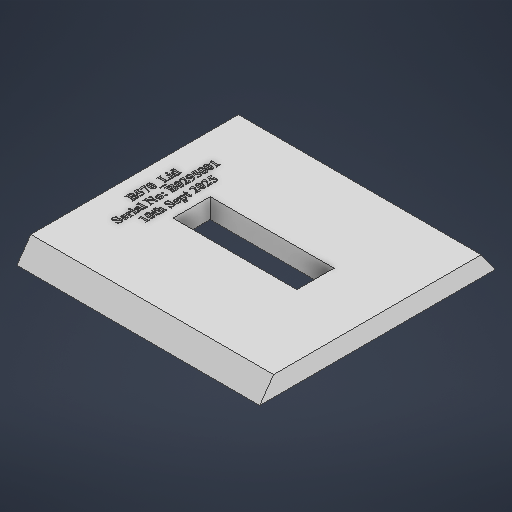
# Autodesk Inventor part: Lid_295
Saved by Autodesk Inventor 2026.1 (Build 301233000, 233)
## iProperties
Created: 2025-09-11
Part Number: Lid_295
Material: Generic
Document SubType Name: Modeling
Designer: usman
Density: 1 g/cm^3
Appearance: Default
Author: usman
Autodesk Inventor part; units mm, degrees
(part 1 of 2)
ref_plane "YZ Plane" through (0, 0, 0) normal (1, 0, 0) x (0, 1, 0)
ref_plane "XZ Plane" through (0, 0, 0) normal (0, 1, 0) x (-1, 0, 0)
ref_plane "XY Plane" through (0, 0, 0) normal (0, 0, 1) x (1, 0, 0)
sketch "Sketch1" plane through (0, 0, 0) normal (1, 0, 0) x (0, 1, 0)
  line L0 (-4, 47.5) -> (4, 47.5)
  line L1 (4, 47.5) -> (4, -47.5)
  line L2 (4, -47.5) -> (-4, -47.5)
  line L3 (-4, -47.5) -> (-4, 47.5)
  line L4 (-4, 47.5) -> (4, -47.5) construction
  line L5 (4, 47.5) -> (-4, -47.5) construction
  line L6 (-4, 47.5) -> (4, 41.8983)
  line L7 (-4, -47.5) -> (4, -41.8983)
  point P0 (0, 0)
  dimension "d0" = 95
  dimension "d1" = 8
  dimension "d2" = 125
  dimension "d3" = 125
  constraints: 16 end point, 2 midpoint, 2 parallel, 2 point on line, 1 horizontal, 1 perpendicular
  measures "d0" distance of L2.end L0.start
  measures "d1" distance of L1.end L2.end
  measures "d2" angle of L1 L6
  measures "d3" angle of L1 L7
extrude "Extrusion1" add sketch "Sketch1" along normal blind 98 contours L6 L1 L7 L3
sketch "Sketch2" plane through (0, 4, 41.8983) normal (0, 1, 0) x (1, 0, 0)
  line L0 (-3.8878, 0.5072) -> (-3.8878, 83.7387) construction
  line L1 (-3.8878, 83.7387) -> (29.5232, 83.7387) construction
  line L2 (29.5232, 83.7387) -> (29.5232, 0.5072) construction
  line L3 (29.5232, 0.5072) -> (-3.8878, 0.5072) construction
  spline S0 degree 2 poles (7.224, 34.2529) (7.3303, 34.7069) (7.4808, 34.891) knots 0 0 0 1 1 1
  spline S1 degree 2 poles (7.4808, 34.891) (7.6935, 35.1556) (8.0333, 35.1556) knots 0 0 0 1 1 1
  spline S2 degree 2 poles (8.0333, 35.1556) (8.3913, 35.1556) (8.6247, 34.8677) knots 0 0 0 1 1 1
  spline S3 degree 2 poles (8.6247, 34.8677) (8.9075, 34.5149) (8.9075, 33.8405) knots 0 0 0 1 1 1
  line L4 (8.9075, 33.8405) -> (8.9075, 32.2244)
  line L5 (8.9075, 32.2244) -> (8.8219, 32.2244)
  spline S4 degree 2 poles (8.8219, 32.2244) (8.8219, 32.4449) (8.7389, 32.6032) (8.6092, 32.6654) (8.3498, 32.6654) knots 0 0 0 1 2 3 3 3
  line L6 (8.3498, 32.6654) -> (6.2902, 32.6654)
  spline S5 degree 2 poles (6.2902, 32.6654) (6.0308, 32.6654) (5.8985, 32.6032) (5.8181, 32.4449) (5.8181, 32.2244) knots 0 0 0 1 2 3 3 3
  line L7 (5.8181, 32.2244) -> (5.7325, 32.2244)
  line L8 (5.7325, 32.2244) -> (5.7325, 33.7471)
  spline S6 degree 2 poles (5.7325, 33.7471) (5.7325, 34.2944) (5.927, 34.7484) (6.3135, 35.0103) (6.5314, 35.0103) knots 0 0 0 1 2 3 3 3
  spline S7 degree 2 poles (6.5314, 35.0103) (6.7597, 35.0103) (7.1202, 34.6757) (7.224, 34.2529) knots 0 0 0 1 2 2 2
  line L9 (7.3433, 33.4047) -> (8.3627, 33.4047)
  line L10 (8.3627, 33.4047) -> (8.4769, 33.4021)
  spline S8 degree 2 poles (8.4769, 33.4021) (8.604, 33.4021) (8.7311, 33.5292) (8.7311, 33.6537) knots 0 0 0 1 2 2 2
  spline S9 degree 2 poles (8.7311, 33.6537) (8.7311, 33.8353) (8.5651, 34.144) (8.2486, 34.31) (8.0567, 34.31) knots 0 0 0 1 2 3 3 3
  spline S10 degree 2 poles (8.0567, 34.31) (7.8336, 34.31) (7.4808, 34.1258) (7.3407, 33.7652) (7.3433, 33.4047) knots 0 0 0 1 2 3 3 3
  spline S11 degree 2 poles (7.1617, 33.4047) (7.1617, 33.7393) (7.0113, 34.0558) (6.7389, 34.2244) (6.5288, 34.2244) knots 0 0 0 1 2 3 3 3
  spline S12 degree 2 poles (6.5288, 34.2244) (6.3161, 34.2244) (6.0463, 34.0584) (5.9063, 33.7471) (5.9089, 33.4047) knots 0 0 0 1 2 3 3 3
  line L11 (5.9089, 33.4047) -> (7.1617, 33.4047)
  line L12 (5.7325, 36.0531) -> (5.7325, 37.5446)
  line L13 (5.7325, 37.5446) -> (6.3369, 37.3086)
  line L14 (6.3369, 37.3086) -> (6.3369, 36.0531)
  line L15 (6.3369, 36.0531) -> (6.6533, 35.9364)
  spline S13 degree 2 poles (6.6533, 35.9364) (6.6845, 36.7457) (7.0554, 37.1815) knots 0 0 0 1 1 1
  spline S14 degree 2 poles (7.0554, 37.1815) (7.3615, 37.5395) (7.818, 37.5395) knots 0 0 0 1 1 1
  spline S15 degree 2 poles (7.818, 37.5395) (8.1111, 37.5395) (8.6714, 37.2074) (8.9723, 36.603) (8.9723, 36.2399) knots 0 0 0 1 2 3 3 3
  spline S16 degree 2 poles (8.9723, 36.2399) (8.9723, 35.8508) (8.8271, 35.6433) knots 0 0 0 1 1 1
  spline S17 degree 2 poles (8.8271, 35.6433) (8.7233, 35.498) (8.5936, 35.498) knots 0 0 0 1 1 1
  spline S18 degree 2 poles (8.5936, 35.498) (8.4924, 35.498) (8.3368, 35.6511) (8.3368, 35.7522) knots 0 0 0 1 2 2 2
  spline S19 degree 2 poles (8.3368, 35.7522) (8.3368, 35.843) (8.412, 36.0298) (8.5728, 36.258) knots 0 0 0 1 2 2 2
  spline S20 degree 2 poles (8.5728, 36.258) (8.6714, 36.4007) (8.7077, 36.5045) knots 0 0 0 1 1 1
  spline S21 degree 2 poles (8.7077, 36.5045) (8.7363, 36.5771) (8.7363, 36.6679) knots 0 0 0 1 1 1
  spline S22 degree 2 poles (8.7363, 36.6679) (8.7363, 36.8598) (8.4561, 37.1296) (8.259, 37.1296) knots 0 0 0 1 2 2 2
  spline S23 degree 2 poles (8.259, 37.1296) (7.8465, 37.1296) (7.3329, 36.3047) (7.3329, 35.6744) knots 0 0 0 1 2 2 2
  spline S24 degree 2 poles (7.3329, 35.6744) (7.3329, 35.6121) (7.3355, 35.485) knots 0 0 0 1 1 1
  line L16 (7.3355, 35.485) -> (5.7325, 36.0531)
  line L17 (8.9723, 38.5744) -> (6.3524, 39.4382)
  line L18 (6.3524, 39.4382) -> (6.3524, 38.7794)
  spline S25 degree 2 poles (6.3524, 38.7794) (6.3524, 38.3929) (6.4536, 38.1983) knots 0 0 0 1 1 1
  spline S26 degree 2 poles (6.4536, 38.1983) (6.5236, 38.0634) (6.7182, 37.9726) knots 0 0 0 1 1 1
  line L19 (6.7182, 37.9726) -> (6.7182, 37.8844)
  line L20 (6.7182, 37.8844) -> (5.7325, 38.1153)
  line L21 (5.7325, 38.1153) -> (5.7325, 40.0115)
  line L22 (5.7325, 40.0115) -> (8.9723, 38.9428)
  line L23 (8.9723, 38.9428) -> (8.9723, 38.5744)
  spline S27 degree 2 poles (7.32, 42.346) (7.7947, 42.346) (8.2071, 42.2138) knots 0 0 0 1 1 1
  spline S28 degree 2 poles (8.2071, 42.2138) (8.4587, 42.1333) (8.783, 41.8636) (8.9723, 41.5212) (8.9723, 41.3214) knots 0 0 0 1 2 3 3 3
  spline S29 degree 2 poles (8.9723, 41.3214) (8.9723, 41.0906) (8.7389, 40.7196) (8.521, 40.577) knots 0 0 0 1 2 2 2
  spline S30 degree 2 poles (8.521, 40.577) (8.3627, 40.4758) (8.0982, 40.398) knots 0 0 0 1 1 1
  spline S31 degree 2 poles (8.0982, 40.398) (7.7376, 40.2968) (7.3563, 40.2968) knots 0 0 0 1 1 1
  spline S32 degree 2 poles (7.3563, 40.2968) (6.8401, 40.2968) (6.4069, 40.4421) knots 0 0 0 1 1 1
  spline S33 degree 2 poles (6.4069, 40.4421) (6.0489, 40.5614) (5.6676, 41.0491) (5.6676, 41.3214) knots 0 0 0 1 2 2 2
  spline S34 degree 2 poles (5.6676, 41.3214) (5.6676, 41.5964) (6.0437, 42.0763) (6.3628, 42.1904) knots 0 0 0 1 2 2 2
  spline S35 degree 2 poles (6.3628, 42.1904) (6.8012, 42.346) (7.32, 42.346) knots 0 0 0 1 1 1
  spline S36 degree 2 poles (7.3148, 41.6249) (6.4821, 41.6249) (6.3446, 41.6146) knots 0 0 0 1 1 1
  spline S37 degree 2 poles (6.3446, 41.6146) (6.0178, 41.5912) (5.9037, 41.503) knots 0 0 0 1 1 1
  spline S38 degree 2 poles (5.9037, 41.503) (5.8284, 41.4459) (5.8284, 41.3137) knots 0 0 0 1 1 1
  spline S39 degree 2 poles (5.8284, 41.3137) (5.8284, 41.2125) (5.8855, 41.1554) knots 0 0 0 1 1 1
  spline S40 degree 2 poles (5.8855, 41.1554) (5.9659, 41.0672) (6.381, 41.0076) (7.6183, 41.0076) knots 0 0 0 1 2 2 2
  spline S41 degree 2 poles (7.6183, 41.0076) (8.2927, 41.0076) (8.5236, 41.0543) knots 0 0 0 1 1 1
  spline S42 degree 2 poles (8.5236, 41.0543) (8.6896, 41.0906) (8.8011, 41.2203) (8.8011, 41.3292) knots 0 0 0 1 2 2 2
  spline S43 degree 2 poles (8.8011, 41.3292) (8.8011, 41.4459) (8.7259, 41.503) knots 0 0 0 1 1 1
  spline S44 degree 2 poles (8.7259, 41.503) (8.5962, 41.6016) (8.3212, 41.6146) knots 0 0 0 1 1 1
  line L24 (8.3212, 41.6146) -> (7.3148, 41.6249)
  line L25 (9.6364, 42.4783) -> (9.6364, 44.9659)
  line L26 (9.6364, 44.9659) -> (9.9425, 44.9659)
  line L27 (9.9425, 44.9659) -> (9.9425, 42.4783)
  line L28 (9.9425, 42.4783) -> (9.6364, 42.4783)
  line L29 (7.7921, 47.949) -> (8.9075, 47.8297)
  line L30 (8.9075, 47.8297) -> (8.9075, 45.0126)
  line L31 (8.9075, 45.0126) -> (8.8219, 45.0126)
  line L32 (8.8219, 45.0126) -> (8.8219, 45.119)
  spline S45 degree 2 poles (8.8219, 45.119) (8.8219, 45.2565) (8.7726, 45.3395) knots 0 0 0 1 1 1
  spline S46 degree 2 poles (8.7726, 45.3395) (8.7389, 45.3991) (8.661, 45.4329) knots 0 0 0 1 1 1
  spline S47 degree 2 poles (8.661, 45.4329) (8.604, 45.4588) (8.3653, 45.4588) knots 0 0 0 1 1 1
  line L33 (8.3653, 45.4588) -> (6.2746, 45.4588)
  spline S48 degree 2 poles (6.2746, 45.4588) (6.0308, 45.4588) (5.9089, 45.4069) (5.8181, 45.2513) (5.8181, 45.119) knots 0 0 0 1 2 3 3 3
  line L34 (5.8181, 45.119) -> (5.8181, 45.0126)
  line L35 (5.8181, 45.0126) -> (5.7325, 45.0126)
  line L36 (5.7325, 45.0126) -> (5.7325, 46.7039)
  line L37 (5.7325, 46.7039) -> (5.8181, 46.7039)
  line L38 (5.8181, 46.7039) -> (5.8181, 46.5664)
  spline S49 degree 2 poles (5.8181, 46.5664) (5.8181, 46.4263) (5.8674, 46.3433) knots 0 0 0 1 1 1
  spline S50 degree 2 poles (5.8674, 46.3433) (5.9011, 46.2811) (5.9789, 46.2474) knots 0 0 0 1 1 1
  spline S51 degree 2 poles (5.9789, 46.2474) (6.036, 46.2214) (6.2746, 46.2214) knots 0 0 0 1 1 1
  line L39 (6.2746, 46.2214) -> (8.2979, 46.2214)
  spline S52 degree 2 poles (8.2979, 46.2214) (8.5417, 46.2214) (8.674, 46.2785) (8.7077, 46.3589) knots 0 0 0 1 2 2 2
  spline S53 degree 2 poles (8.7077, 46.3589) (8.7285, 46.4186) (8.7285, 46.6416) knots 0 0 0 1 1 1
  line L40 (8.7285, 46.6416) -> (8.7285, 46.9062)
  spline S54 degree 2 poles (8.7285, 46.9062) (8.7285, 47.1604) (8.5495, 47.4976) (8.1656, 47.7441) (7.7921, 47.853) knots 0 0 0 1 2 3 3 3
  line L41 (7.7921, 47.853) -> (7.7921, 47.949)
  line L42 (6.7182, 49.137) -> (8.4535, 49.137)
  spline S55 degree 2 poles (8.4535, 49.137) (8.687, 49.137) (8.8141, 49.246) (8.8245, 49.4042) knots 0 0 0 1 2 2 2
  line L43 (8.8245, 49.4042) -> (8.9075, 49.4042)
  line L44 (8.9075, 49.4042) -> (8.9075, 48.2188)
  line L45 (8.9075, 48.2188) -> (8.8245, 48.2188)
  spline S56 degree 2 poles (8.8245, 48.2188) (8.8193, 48.364) (8.7389, 48.4341) knots 0 0 0 1 1 1
  spline S57 degree 2 poles (8.7389, 48.4341) (8.687, 48.4807) (8.4535, 48.4807) knots 0 0 0 1 1 1
  line L46 (8.4535, 48.4807) -> (7.1747, 48.4807)
  spline S58 degree 2 poles (7.1747, 48.4807) (6.9413, 48.4807) (6.8141, 48.3744) (6.8038, 48.2188) knots 0 0 0 1 2 2 2
  line L47 (6.8038, 48.2188) -> (6.7182, 48.2188)
  line L48 (6.7182, 48.2188) -> (6.7182, 49.137)
  spline S59 degree 2 poles (5.6598, 48.8102) (5.6598, 48.9632) (5.8725, 49.1733) (6.023, 49.1733) knots 0 0 0 1 2 2 2
  spline S60 degree 2 poles (6.023, 49.1733) (6.1734, 49.1733) (6.3836, 48.9606) (6.3836, 48.8102) knots 0 0 0 1 2 2 2
  spline S61 degree 2 poles (6.3836, 48.8102) (6.3836, 48.6597) (6.1734, 48.4496) (6.023, 48.4496) knots 0 0 0 1 2 2 2
  spline S62 degree 2 poles (6.023, 48.4496) (5.8725, 48.4496) (5.6598, 48.6597) (5.6598, 48.8102) knots 0 0 0 1 2 2 2
  line L49 (5.7325, 51.7439) -> (8.2512, 51.7439)
  spline S63 degree 2 poles (8.2512, 51.7439) (8.508, 51.7439) (8.5547, 51.7569) knots 0 0 0 1 1 1
  spline S64 degree 2 poles (8.5547, 51.7569) (8.6299, 51.7777) (8.7051, 51.8814) (8.7155, 52.0111) knots 0 0 0 1 2 2 2
  line L50 (8.7155, 52.0111) -> (8.7933, 52.0111)
  line L51 (8.7933, 52.0111) -> (8.9723, 51.0877)
  line L52 (8.9723, 51.0877) -> (8.6247, 51.0877)
  spline S65 degree 2 poles (8.6247, 51.0877) (8.8271, 50.9217) (8.9723, 50.6623) (8.9723, 50.4963) knots 0 0 0 1 2 2 2
  spline S66 degree 2 poles (8.9723, 50.4963) (8.9723, 50.0786) (8.5988, 49.8348) knots 0 0 0 1 1 1
  spline S67 degree 2 poles (8.5988, 49.8348) (8.2927, 49.6377) (7.8517, 49.6377) knots 0 0 0 1 1 1
  spline S68 degree 2 poles (7.8517, 49.6377) (7.499, 49.6377) (6.9387, 49.8815) (6.6533, 50.3043) (6.6533, 50.5481) knots 0 0 0 1 2 3 3 3
  spline S69 degree 2 poles (6.6533, 50.5481) (6.6533, 50.7064) (6.7752, 50.9502) (6.9283, 51.0877) knots 0 0 0 1 2 2 2
  line L53 (6.9283, 51.0877) -> (6.2668, 51.0877)
  spline S70 degree 2 poles (6.2668, 51.0877) (6.0152, 51.0877) (5.9633, 51.0669) knots 0 0 0 1 1 1
  spline S71 degree 2 poles (5.9633, 51.0669) (5.8959, 51.0384) (5.831, 50.9268) (5.831, 50.7712) knots 0 0 0 1 2 2 2
  line L54 (5.831, 50.7712) -> (5.7325, 50.7712)
  line L55 (5.7325, 50.7712) -> (5.7325, 51.7439)
  spline S72 degree 2 poles (7.2188, 51.0877) (6.8842, 50.9139) (6.8842, 50.6649) knots 0 0 0 1 1 1
  spline S73 degree 2 poles (6.8842, 50.6649) (6.8842, 50.5767) (6.9309, 50.5222) knots 0 0 0 1 1 1
  spline S74 degree 2 poles (6.9309, 50.5222) (7.0035, 50.434) (7.3693, 50.3251) (7.7454, 50.3251) knots 0 0 0 1 2 2 2
  spline S75 degree 2 poles (7.7454, 50.3251) (8.1604, 50.3251) (8.5599, 50.447) (8.6481, 50.5507) knots 0 0 0 1 2 2 2
  spline S76 degree 2 poles (8.6481, 50.5507) (8.6922, 50.6052) (8.6922, 50.6986) knots 0 0 0 1 1 1
  spline S77 degree 2 poles (8.6922, 50.6986) (8.6922, 50.9061) (8.3705, 51.0877) knots 0 0 0 1 1 1
  line L56 (8.3705, 51.0877) -> (7.2188, 51.0877)
  line L57 (10.6816, 23.453) -> (11.7399, 23.4789)
  line L58 (11.7399, 23.4789) -> (11.7399, 23.3829)
  spline S78 degree 2 poles (11.7399, 23.3829) (11.343, 23.3155) (10.8579, 22.7811) (10.8579, 22.4725) knots 0 0 0 1 2 2 2
  spline S79 degree 2 poles (10.8579, 22.4725) (10.8579, 22.2338) (11.1121, 21.9537) (11.2782, 21.9537) knots 0 0 0 1 2 2 2
  spline S80 degree 2 poles (11.2782, 21.9537) (11.3845, 21.9537) (11.4649, 22.003) knots 0 0 0 1 1 1
  spline S81 degree 2 poles (11.4649, 22.003) (11.5765, 22.0704) (11.6828, 22.2209) knots 0 0 0 1 1 1
  spline S82 degree 2 poles (11.6828, 22.2209) (11.7606, 22.3324) (11.9578, 22.7319) knots 0 0 0 1 1 1
  spline S83 degree 2 poles (11.9578, 22.7319) (12.2301, 23.2896) (12.474, 23.4841) knots 0 0 0 1 1 1
  spline S84 degree 2 poles (12.474, 23.4841) (12.7178, 23.6761) (13.0317, 23.6761) knots 0 0 0 1 1 1
  spline S85 degree 2 poles (13.0317, 23.6761) (13.4286, 23.6761) (14.0018, 23.0561) (14.0018, 22.5762) knots 0 0 0 1 2 2 2
  spline S86 degree 2 poles (14.0018, 22.5762) (14.0018, 22.4258) (13.9422, 22.1586) (13.8566, 21.9589) knots 0 0 0 1 2 2 2
  spline S87 degree 2 poles (13.8566, 21.9589) (13.8099, 21.8447) (13.8099, 21.7721) knots 0 0 0 1 1 1
  spline S88 degree 2 poles (13.8099, 21.7721) (13.8099, 21.7124) (13.9058, 21.575) (14.0018, 21.5335) knots 0 0 0 1 2 2 2
  line L59 (14.0018, 21.5335) -> (14.0018, 21.4479)
  line L60 (14.0018, 21.4479) -> (12.8034, 21.4479)
  line L61 (12.8034, 21.4479) -> (12.8034, 21.5335)
  spline S89 degree 2 poles (12.8034, 21.5335) (13.3092, 21.6372) (13.8384, 22.226) (13.8384, 22.5658) knots 0 0 0 1 2 2 2
  spline S90 degree 2 poles (13.8384, 22.5658) (13.8384, 22.8278) (13.5531, 23.1391) (13.3637, 23.1391) knots 0 0 0 1 2 2 2
  spline S91 degree 2 poles (13.3637, 23.1391) (13.2522, 23.1391) (13.0395, 23.0198) (12.8501, 22.776) (12.6996, 22.4647) knots 0 0 0 1 2 3 3 3
  spline S92 degree 2 poles (12.6996, 22.4647) (12.4869, 22.0315) (12.186, 21.6528) (11.8177, 21.4504) (11.5946, 21.4504) knots 0 0 0 1 2 3 3 3
  spline S93 degree 2 poles (11.5946, 21.4504) (11.2159, 21.4504) (10.6816, 22.0081) (10.6816, 22.431) knots 0 0 0 1 2 2 2
  spline S94 degree 2 poles (10.6816, 22.431) (10.6816, 22.5866) (10.7179, 22.7319) knots 0 0 0 1 1 1
  spline S95 degree 2 poles (10.7179, 22.7319) (10.7464, 22.8408) (10.8994, 23.1573) (10.8994, 23.2221) knots 0 0 0 1 2 2 2
  spline S96 degree 2 poles (10.8994, 23.2221) (10.8994, 23.2818) (10.8242, 23.3518) (10.6816, 23.3829) knots 0 0 0 1 2 2 2
  line L62 (10.6816, 23.3829) -> (10.6816, 23.453)
  line L63 (12.7593, 25.8861) -> (12.7593, 24.6825)
  spline S97 degree 2 poles (12.7593, 24.6825) (13.1925, 24.7033) (13.4441, 24.916) knots 0 0 0 1 1 1
  spline S98 degree 2 poles (13.4441, 24.916) (13.6387, 25.0768) (13.6387, 25.3051) knots 0 0 0 1 1 1
  spline S99 degree 2 poles (13.6387, 25.3051) (13.6387, 25.4451) (13.483, 25.676) (13.2781, 25.8057) knots 0 0 0 1 2 2 2
  line L64 (13.2781, 25.8057) -> (13.33, 25.8861)
  spline S100 degree 2 poles (13.33, 25.8861) (13.6931, 25.7071) (13.994, 25.2765) (13.994, 24.9938) knots 0 0 0 1 2 2 2
  spline S101 degree 2 poles (13.994, 24.9938) (13.994, 24.5035) (13.6205, 24.2545) knots 0 0 0 1 1 1
  spline S102 degree 2 poles (13.6205, 24.2545) (13.317, 24.0522) (12.8709, 24.0522) knots 0 0 0 1 1 1
  spline S103 degree 2 poles (12.8709, 24.0522) (12.3235, 24.0522) (11.675, 24.6462) (11.675, 25.0431) knots 0 0 0 1 2 2 2
  spline S104 degree 2 poles (11.675, 25.0431) (11.675, 25.3777) (12.2224, 25.868) (12.7593, 25.8861) knots 0 0 0 1 2 2 2
  spline S105 degree 2 poles (12.6011, 25.3103) (12.225, 25.3103) (11.9422, 25.2272) (11.8696, 25.1416) knots 0 0 0 1 2 2 2
  spline S106 degree 2 poles (11.8696, 25.1416) (11.8281, 25.0924) (11.8281, 25.0094) knots 0 0 0 1 1 1
  spline S107 degree 2 poles (11.8281, 25.0094) (11.8281, 24.8874) (11.9474, 24.8096) knots 0 0 0 1 1 1
  spline S108 degree 2 poles (11.9474, 24.8096) (12.1549, 24.6721) (12.5181, 24.6721) knots 0 0 0 1 1 1
  line L65 (12.5181, 24.6721) -> (12.6011, 24.6721)
  line L66 (12.6011, 24.6721) -> (12.6011, 25.3103)
  line L67 (11.7399, 27.0715) -> (12.2353, 27.0715)
  spline S109 degree 2 poles (12.2353, 27.0715) (11.8981, 27.2894) (11.675, 27.6163) (11.675, 27.7693) knots 0 0 0 1 2 2 2
  spline S110 degree 2 poles (11.675, 27.7693) (11.675, 27.899) (11.8359, 28.0547) (11.9837, 28.0547) knots 0 0 0 1 2 2 2
  spline S111 degree 2 poles (11.9837, 28.0547) (12.1394, 28.0547) (12.3132, 27.9016) (12.3132, 27.7953) knots 0 0 0 1 2 2 2
  spline S112 degree 2 poles (12.3132, 27.7953) (12.3132, 27.6733) (12.1549, 27.4918) (12.1445, 27.4762) knots 0 0 0 1 2 2 2
  spline S113 degree 2 poles (12.1445, 27.4762) (12.1316, 27.4529) (12.1316, 27.4217) knots 0 0 0 1 1 1
  spline S114 degree 2 poles (12.1316, 27.4217) (12.1316, 27.3543) (12.1835, 27.292) knots 0 0 0 1 1 1
  spline S115 degree 2 poles (12.1835, 27.292) (12.2613, 27.1961) (12.4091, 27.1494) knots 0 0 0 1 1 1
  spline S116 degree 2 poles (12.4091, 27.1494) (12.6374, 27.0741) (12.9098, 27.0741) knots 0 0 0 1 1 1
  line L68 (12.9098, 27.0741) -> (13.413, 27.0741)
  line L69 (13.413, 27.0741) -> (13.5453, 27.0741)
  spline S117 degree 2 poles (13.5453, 27.0741) (13.6802, 27.0741) (13.7165, 27.0897) knots 0 0 0 1 1 1
  spline S118 degree 2 poles (13.7165, 27.0897) (13.7813, 27.1182) (13.8384, 27.2298) (13.8462, 27.3595) knots 0 0 0 1 2 2 2
  line L70 (13.8462, 27.3595) -> (13.9292, 27.3595)
  line L71 (13.9292, 27.3595) -> (13.9292, 26.174)
  line L72 (13.9292, 26.174) -> (13.8462, 26.174)
  spline S119 degree 2 poles (13.8462, 26.174) (13.8332, 26.3167) (13.7009, 26.4179) (13.413, 26.4179) knots 0 0 0 1 2 2 2
  line L73 (13.413, 26.4179) -> (12.2042, 26.4179)
  spline S120 degree 2 poles (12.2042, 26.4179) (12.0148, 26.4179) (11.963, 26.3997) knots 0 0 0 1 1 1
  spline S121 degree 2 poles (11.963, 26.3997) (11.8981, 26.3764) (11.8385, 26.2856) (11.8255, 26.174) knots 0 0 0 1 2 2 2
  line L74 (11.8255, 26.174) -> (11.7399, 26.174)
  line L75 (11.7399, 26.174) -> (11.7399, 27.0715)
  line L76 (11.7399, 29.1441) -> (13.4752, 29.1441)
  spline S122 degree 2 poles (13.4752, 29.1441) (13.7087, 29.1441) (13.8358, 29.2531) (13.8462, 29.4113) knots 0 0 0 1 2 2 2
  line L77 (13.8462, 29.4113) -> (13.9292, 29.4113)
  line L78 (13.9292, 29.4113) -> (13.9292, 28.2259)
  line L79 (13.9292, 28.2259) -> (13.8462, 28.2259)
  spline S123 degree 2 poles (13.8462, 28.2259) (13.841, 28.3711) (13.7606, 28.4412) knots 0 0 0 1 1 1
  spline S124 degree 2 poles (13.7606, 28.4412) (13.7087, 28.4878) (13.4752, 28.4878) knots 0 0 0 1 1 1
  line L80 (13.4752, 28.4878) -> (12.1964, 28.4878)
  spline S125 degree 2 poles (12.1964, 28.4878) (11.963, 28.4878) (11.8359, 28.3815) (11.8255, 28.2259) knots 0 0 0 1 2 2 2
  line L81 (11.8255, 28.2259) -> (11.7399, 28.2259)
  line L82 (11.7399, 28.2259) -> (11.7399, 29.1441)
  spline S126 degree 2 poles (10.6816, 28.8173) (10.6816, 28.9703) (10.8943, 29.1804) (11.0447, 29.1804) knots 0 0 0 1 2 2 2
  spline S127 degree 2 poles (11.0447, 29.1804) (11.1952, 29.1804) (11.4053, 28.9677) (11.4053, 28.8173) knots 0 0 0 1 2 2 2
  spline S128 degree 2 poles (11.4053, 28.8173) (11.4053, 28.6668) (11.1952, 28.4567) (11.0447, 28.4567) knots 0 0 0 1 2 2 2
  spline S129 degree 2 poles (11.0447, 28.4567) (10.8943, 28.4567) (10.6816, 28.6668) (10.6816, 28.8173) knots 0 0 0 1 2 2 2
  spline S130 degree 2 poles (13.6075, 30.8328) (13.9603, 30.4307) (13.9603, 30.1117) knots 0 0 0 1 1 1
  spline S131 degree 2 poles (13.9603, 30.1117) (13.9603, 29.9249) (13.7139, 29.6759) (13.5297, 29.6759) knots 0 0 0 1 2 2 2
  spline S132 degree 2 poles (13.5297, 29.6759) (13.2781, 29.6759) (12.8786, 30.1065) (12.544, 30.8328) knots 0 0 0 1 2 2 2
  line L83 (12.544, 30.8328) -> (12.3261, 30.8328)
  spline S133 degree 2 poles (12.3261, 30.8328) (12.0771, 30.8328) (11.95, 30.7783) (11.854, 30.6279) (11.854, 30.5345) knots 0 0 0 1 2 3 3 3
  spline S134 degree 2 poles (11.854, 30.5345) (11.854, 30.3814) (11.9215, 30.2829) knots 0 0 0 1 1 1
  spline S135 degree 2 poles (11.9215, 30.2829) (11.963, 30.2206) (12.02, 30.2206) knots 0 0 0 1 1 1
  spline S136 degree 2 poles (12.02, 30.2206) (12.0693, 30.2206) (12.1419, 30.2881) knots 0 0 0 1 1 1
  spline S137 degree 2 poles (12.1419, 30.2881) (12.2431, 30.3762) (12.3365, 30.3762) knots 0 0 0 1 1 1
  spline S138 degree 2 poles (12.3365, 30.3762) (12.4506, 30.3762) (12.6115, 30.205) (12.6115, 30.0676) knots 0 0 0 1 2 2 2
  spline S139 degree 2 poles (12.6115, 30.0676) (12.6115, 29.9197) (12.4325, 29.72) (12.3132, 29.72) knots 0 0 0 1 2 2 2
  spline S140 degree 2 poles (12.3132, 29.72) (12.1445, 29.72) (11.8385, 29.9872) (11.675, 30.467) (11.675, 30.7238) knots 0 0 0 1 2 3 3 3
  spline S141 degree 2 poles (11.675, 30.7238) (11.675, 31.0351) (11.9396, 31.4009) (12.0927, 31.4527) knots 0 0 0 1 2 2 2
  spline S142 degree 2 poles (12.0927, 31.4527) (12.1912, 31.4865) (12.5466, 31.4865) knots 0 0 0 1 1 1
  line L84 (12.5466, 31.4865) -> (13.3948, 31.4865)
  spline S143 degree 2 poles (13.3948, 31.4865) (13.5453, 31.4865) (13.6231, 31.5098) (13.6594, 31.5565) (13.6594, 31.5876) knots 0 0 0 1 2 3 3 3
  spline S144 degree 2 poles (13.6594, 31.5876) (13.6594, 31.6499) (13.5738, 31.7121) knots 0 0 0 1 1 1
  line L85 (13.5738, 31.7121) -> (13.6283, 31.7822)
  spline S145 degree 2 poles (13.6283, 31.7822) (13.8021, 31.6654) (13.9603, 31.4138) (13.9603, 31.2556) knots 0 0 0 1 2 2 2
  spline S146 degree 2 poles (13.9603, 31.2556) (13.9603, 31.0662) (13.7839, 30.8561) (13.6075, 30.8328) knots 0 0 0 1 2 2 2
  line L86 (13.4363, 30.8328) -> (12.7022, 30.8328)
  spline S147 degree 2 poles (12.7022, 30.8328) (12.8683, 30.5474) (13.0576, 30.4074) knots 0 0 0 1 1 1
  spline S148 degree 2 poles (13.0576, 30.4074) (13.1847, 30.3166) (13.3144, 30.3166) knots 0 0 0 1 1 1
  spline S149 degree 2 poles (13.3144, 30.3166) (13.4208, 30.3166) (13.5038, 30.3944) knots 0 0 0 1 1 1
  spline S150 degree 2 poles (13.5038, 30.3944) (13.566, 30.4541) (13.566, 30.5604) knots 0 0 0 1 1 1
  spline S151 degree 2 poles (13.566, 30.5604) (13.566, 30.6771) (13.4363, 30.8328) knots 0 0 0 1 1 1
  line L87 (10.7542, 32.8794) -> (13.4752, 32.8794)
  spline S152 degree 2 poles (13.4752, 32.8794) (13.7087, 32.8794) (13.8358, 32.9884) (13.8462, 33.1466) knots 0 0 0 1 2 2 2
  line L88 (13.8462, 33.1466) -> (13.9292, 33.1466)
  line L89 (13.9292, 33.1466) -> (13.9292, 31.9612)
  line L90 (13.9292, 31.9612) -> (13.8462, 31.9612)
  spline S153 degree 2 poles (13.8462, 31.9612) (13.841, 32.1064) (13.7606, 32.1765) knots 0 0 0 1 1 1
  spline S154 degree 2 poles (13.7606, 32.1765) (13.7087, 32.2231) (13.4752, 32.2231) knots 0 0 0 1 1 1
  line L91 (13.4752, 32.2231) -> (11.2081, 32.2231)
  spline S155 degree 2 poles (11.2081, 32.2231) (10.9773, 32.2231) (10.8502, 32.1168) (10.8398, 31.9612) knots 0 0 0 1 2 2 2
  line L92 (10.8398, 31.9612) -> (10.7542, 31.9612)
  line L93 (10.7542, 31.9612) -> (10.7542, 32.8794)
  line L94 (10.7542, 35.5849) -> (12.723, 37.1517)
  line L95 (12.723, 37.1517) -> (11.3586, 37.1517)
  spline S156 degree 2 poles (11.3586, 37.1517) (11.0732, 37.1517) (10.9721, 37.0686) knots 0 0 0 1 1 1
  spline S157 degree 2 poles (10.9721, 37.0686) (10.8346, 36.9571) (10.8398, 36.6925) knots 0 0 0 1 1 1
  line L96 (10.8398, 36.6925) -> (10.7542, 36.6925)
  line L97 (10.7542, 36.6925) -> (10.7542, 37.7431)
  line L98 (10.7542, 37.7431) -> (10.8398, 37.7431)
  spline S158 degree 2 poles (10.8398, 37.7431) (10.8657, 37.5407) (10.9487, 37.4033) (11.1329, 37.3254) (11.3586, 37.3254) knots 0 0 0 1 2 3 3 3
  line L99 (11.3586, 37.3254) -> (14.0018, 37.3254)
  line L100 (14.0018, 37.3254) -> (14.0018, 37.245)
  line L101 (14.0018, 37.245) -> (11.356, 35.0972)
  line L102 (11.356, 35.0972) -> (13.3767, 35.0972)
  spline S159 degree 2 poles (13.3767, 35.0972) (13.6516, 35.0972) (13.8436, 35.3489) (13.8436, 35.5097) knots 0 0 0 1 2 2 2
  line L103 (13.8436, 35.5097) -> (13.8436, 35.5849)
  line L104 (13.8436, 35.5849) -> (13.9292, 35.5849)
  line L105 (13.9292, 35.5849) -> (13.9292, 34.4565)
  line L106 (13.9292, 34.4565) -> (13.8436, 34.4565)
  spline S160 degree 2 poles (13.8436, 34.4565) (13.841, 34.7185) (13.6309, 34.926) (13.3767, 34.926) knots 0 0 0 1 2 2 2
  line L107 (13.3767, 34.926) -> (11.1355, 34.926)
  line L108 (11.1355, 34.926) -> (11.0525, 34.8586)
  spline S161 degree 2 poles (11.0525, 34.8586) (10.9254, 34.7574) (10.845, 34.6044) (10.8398, 34.4591) knots 0 0 0 1 2 2 2
  line L109 (10.8398, 34.4591) -> (10.7542, 34.4591)
  line L110 (10.7542, 34.4591) -> (10.7542, 35.5849)
  spline S162 degree 2 poles (11.675, 39.0504) (11.675, 39.3358) (11.9707, 39.826) (12.5129, 40.0802) (12.8345, 40.0802) knots 0 0 0 1 2 3 3 3
  spline S163 degree 2 poles (12.8345, 40.0802) (13.3014, 40.0802) (13.6153, 39.8442) knots 0 0 0 1 1 1
  spline S164 degree 2 poles (13.6153, 39.8442) (13.994, 39.5588) (13.994, 39.0556) knots 0 0 0 1 1 1
  spline S165 degree 2 poles (13.994, 39.0556) (13.994, 38.5628) (13.3014, 38.031) (12.8449, 38.031) knots 0 0 0 1 2 2 2
  spline S166 degree 2 poles (12.8449, 38.031) (12.3754, 38.031) (11.675, 38.5757) (11.675, 39.0504) knots 0 0 0 1 2 2 2
  spline S167 degree 2 poles (11.8411, 39.0608) (11.8411, 38.9415) (12.02, 38.7729) (12.5518, 38.7184) (13.0265, 38.7184) knots 0 0 0 1 2 3 3 3
  spline S168 degree 2 poles (13.0265, 38.7184) (13.2755, 38.7184) (13.4934, 38.7521) knots 0 0 0 1 1 1
  spline S169 degree 2 poles (13.4934, 38.7521) (13.6594, 38.7755) (13.8332, 38.9441) (13.8332, 39.0504) knots 0 0 0 1 2 2 2
  spline S170 degree 2 poles (13.8332, 39.0504) (13.8332, 39.1568) (13.7735, 39.2242) knots 0 0 0 1 1 1
  spline S171 degree 2 poles (13.7735, 39.2242) (13.6957, 39.315) (13.5531, 39.3461) knots 0 0 0 1 1 1
  spline S172 degree 2 poles (13.5531, 39.3461) (13.33, 39.3928) (12.653, 39.3928) knots 0 0 0 1 1 1
  spline S173 degree 2 poles (12.653, 39.3928) (12.2561, 39.3928) (11.9578, 39.3046) (11.8903, 39.219) knots 0 0 0 1 2 2 2
  spline S174 degree 2 poles (11.8903, 39.219) (11.8411, 39.1568) (11.8411, 39.0608) knots 0 0 0 1 1 1
  spline S175 degree 2 poles (13.2081, 41.0556) (13.2081, 41.219) (13.4389, 41.4472) (13.5998, 41.4472) knots 0 0 0 1 2 2 2
  spline S176 degree 2 poles (13.5998, 41.4472) (13.7606, 41.4472) (13.9888, 41.2164) (13.9888, 41.0556) knots 0 0 0 1 2 2 2
  spline S177 degree 2 poles (13.9888, 41.0556) (13.9888, 40.8921) (13.7606, 40.6639) (13.5998, 40.6639) knots 0 0 0 1 2 2 2
  spline S178 degree 2 poles (13.5998, 40.6639) (13.4389, 40.6639) (13.2081, 40.8921) (13.2081, 41.0556) knots 0 0 0 1 2 2 2
  spline S179 degree 2 poles (11.675, 41.0581) (11.675, 41.219) (11.9033, 41.4472) (12.0641, 41.4472) knots 0 0 0 1 2 2 2
  spline S180 degree 2 poles (12.0641, 41.4472) (12.225, 41.4472) (12.4532, 41.219) (12.4532, 41.0581) knots 0 0 0 1 2 2 2
  spline S181 degree 2 poles (12.4532, 41.0581) (12.4532, 40.8973) (12.225, 40.6691) (12.0641, 40.6691) knots 0 0 0 1 2 2 2
  spline S182 degree 2 poles (12.0641, 40.6691) (11.9033, 40.6691) (11.675, 40.8973) (11.675, 41.0581) knots 0 0 0 1 2 2 2
  spline S183 degree 2 poles (12.2457, 45.1773) (12.3521, 45.6313) (12.5025, 45.8155) knots 0 0 0 1 1 1
  spline S184 degree 2 poles (12.5025, 45.8155) (12.7152, 46.08) (13.055, 46.08) knots 0 0 0 1 1 1
  spline S185 degree 2 poles (13.055, 46.08) (13.413, 46.08) (13.6464, 45.7921) knots 0 0 0 1 1 1
  spline S186 degree 2 poles (13.6464, 45.7921) (13.9292, 45.4393) (13.9292, 44.7649) knots 0 0 0 1 1 1
  line L111 (13.9292, 44.7649) -> (13.9292, 43.1489)
  line L112 (13.9292, 43.1489) -> (13.8436, 43.1489)
  spline S187 degree 2 poles (13.8436, 43.1489) (13.8436, 43.3694) (13.7606, 43.5276) (13.6309, 43.5898) (13.3715, 43.5898) knots 0 0 0 1 2 3 3 3
  line L113 (13.3715, 43.5898) -> (11.3119, 43.5898)
  spline S188 degree 2 poles (11.3119, 43.5898) (11.0525, 43.5898) (10.9202, 43.5276) (10.8398, 43.3694) (10.8398, 43.1489) knots 0 0 0 1 2 3 3 3
  line L114 (10.8398, 43.1489) -> (10.7542, 43.1489)
  line L115 (10.7542, 43.1489) -> (10.7542, 44.6715)
  spline S189 degree 2 poles (10.7542, 44.6715) (10.7542, 45.2189) (10.9487, 45.6728) (11.3352, 45.9348) (11.5531, 45.9348) knots 0 0 0 1 2 3 3 3
  spline S190 degree 2 poles (11.5531, 45.9348) (11.7814, 45.9348) (12.1419, 45.6002) (12.2457, 45.1773) knots 0 0 0 1 2 2 2
  line L116 (12.365, 44.3291) -> (13.3845, 44.3291)
  line L117 (13.3845, 44.3291) -> (13.4986, 44.3265)
  spline S191 degree 2 poles (13.4986, 44.3265) (13.6257, 44.3265) (13.7528, 44.4536) (13.7528, 44.5781) knots 0 0 0 1 2 2 2
  spline S192 degree 2 poles (13.7528, 44.5781) (13.7528, 44.7597) (13.5868, 45.0684) (13.2703, 45.2344) (13.0784, 45.2344) knots 0 0 0 1 2 3 3 3
  spline S193 degree 2 poles (13.0784, 45.2344) (12.8553, 45.2344) (12.5025, 45.0502) (12.3624, 44.6897) (12.365, 44.3291) knots 0 0 0 1 2 3 3 3
  spline S194 degree 2 poles (12.1835, 44.3291) (12.1835, 44.6637) (12.033, 44.9802) (11.7606, 45.1488) (11.5505, 45.1488) knots 0 0 0 1 2 3 3 3
  spline S195 degree 2 poles (11.5505, 45.1488) (11.3378, 45.1488) (11.0681, 44.9828) (10.928, 44.6715) (10.9306, 44.3291) knots 0 0 0 1 2 3 3 3
  line L118 (10.9306, 44.3291) -> (12.1835, 44.3291)
  spline S196 degree 2 poles (12.3417, 48.4717) (12.8164, 48.4717) (13.2288, 48.3394) knots 0 0 0 1 1 1
  spline S197 degree 2 poles (13.2288, 48.3394) (13.4804, 48.259) (13.8047, 47.9892) (13.994, 47.6468) (13.994, 47.4471) knots 0 0 0 1 2 3 3 3
  spline S198 degree 2 poles (13.994, 47.4471) (13.994, 47.2162) (13.7606, 46.8453) (13.5427, 46.7026) knots 0 0 0 1 2 2 2
  spline S199 degree 2 poles (13.5427, 46.7026) (13.3845, 46.6014) (13.1199, 46.5236) knots 0 0 0 1 1 1
  spline S200 degree 2 poles (13.1199, 46.5236) (12.7593, 46.4224) (12.378, 46.4224) knots 0 0 0 1 1 1
  spline S201 degree 2 poles (12.378, 46.4224) (11.8618, 46.4224) (11.4286, 46.5677) knots 0 0 0 1 1 1
  spline S202 degree 2 poles (11.4286, 46.5677) (11.0706, 46.687) (10.6893, 47.1747) (10.6893, 47.4471) knots 0 0 0 1 2 2 2
  spline S203 degree 2 poles (10.6893, 47.4471) (10.6893, 47.722) (11.0655, 48.2019) (11.3845, 48.316) knots 0 0 0 1 2 2 2
  spline S204 degree 2 poles (11.3845, 48.316) (11.8229, 48.4717) (12.3417, 48.4717) knots 0 0 0 1 1 1
  spline S205 degree 2 poles (12.3365, 47.7506) (11.5038, 47.7506) (11.3664, 47.7402) knots 0 0 0 1 1 1
  spline S206 degree 2 poles (11.3664, 47.7402) (11.0395, 47.7168) (10.9254, 47.6286) knots 0 0 0 1 1 1
  spline S207 degree 2 poles (10.9254, 47.6286) (10.8502, 47.5716) (10.8502, 47.4393) knots 0 0 0 1 1 1
  spline S208 degree 2 poles (10.8502, 47.4393) (10.8502, 47.3381) (10.9072, 47.281) knots 0 0 0 1 1 1
  spline S209 degree 2 poles (10.9072, 47.281) (10.9876, 47.1929) (11.4027, 47.1332) (12.64, 47.1332) knots 0 0 0 1 2 2 2
  spline S210 degree 2 poles (12.64, 47.1332) (13.3144, 47.1332) (13.5453, 47.1799) knots 0 0 0 1 1 1
  spline S211 degree 2 poles (13.5453, 47.1799) (13.7113, 47.2162) (13.8228, 47.3459) (13.8228, 47.4548) knots 0 0 0 1 2 2 2
  spline S212 degree 2 poles (13.8228, 47.4548) (13.8228, 47.5716) (13.7476, 47.6286) knots 0 0 0 1 1 1
  spline S213 degree 2 poles (13.7476, 47.6286) (13.6179, 47.7272) (13.343, 47.7402) knots 0 0 0 1 1 1
  line L119 (13.343, 47.7402) -> (12.3365, 47.7506)
  line L120 (13.9292, 50.635) -> (13.9292, 48.7648)
  line L121 (13.9292, 48.7648) -> (13.8773, 48.7648)
  spline S214 degree 2 poles (13.8773, 48.7648) (12.8553, 49.6286) (12.1471, 49.9943) (11.8099, 49.9943) knots 0 0 0 1 2 2 2
  spline S215 degree 2 poles (11.8099, 49.9943) (11.5635, 49.9943) (11.2393, 49.6882) (11.2393, 49.4677) knots 0 0 0 1 2 2 2
  spline S216 degree 2 poles (11.2393, 49.4677) (11.2393, 49.1072) (11.5998, 48.9075) knots 0 0 0 1 1 1
  line L122 (11.5998, 48.9075) -> (11.5687, 48.8219)
  spline S217 degree 2 poles (11.5687, 48.8219) (11.1199, 48.949) (10.6893, 49.4626) (10.6893, 49.8024) knots 0 0 0 1 2 2 2
  spline S218 degree 2 poles (10.6893, 49.8024) (10.6893, 50.0436) (10.915, 50.4405) (11.3041, 50.6662) (11.4753, 50.6662) knots 0 0 0 1 2 3 3 3
  spline S219 degree 2 poles (11.4753, 50.6662) (11.7866, 50.6662) (12.1082, 50.4924) knots 0 0 0 1 1 1
  spline S220 degree 2 poles (12.1082, 50.4924) (12.5388, 50.2563) (13.3144, 49.46) knots 0 0 0 1 1 1
  line L123 (13.3144, 49.46) -> (13.3144, 50.1448)
  spline S221 degree 2 poles (13.3144, 50.1448) (13.3144, 50.399) (13.2729, 50.552) (13.1717, 50.6506) (13.0109, 50.7284) knots 0 0 0 1 2 3 3 3
  line L124 (13.0109, 50.7284) -> (13.0109, 50.814)
  line L125 (13.0109, 50.814) -> (13.9292, 50.635)
  line L126 (13.994, 51.1953) -> (13.9292, 51.1953)
  spline S222 degree 2 poles (13.9292, 51.1953) (13.841, 51.5844) (13.4934, 52.1266) (12.9824, 52.443) (12.6504, 52.5053) knots 0 0 0 1 2 3 3 3
  spline S223 degree 2 poles (12.6504, 52.5053) (12.7256, 52.36) (12.7827, 52.1577) (12.7827, 52.0435) knots 0 0 0 1 2 2 2
  spline S224 degree 2 poles (12.7827, 52.0435) (12.7827, 51.683) (12.2639, 51.2031) (11.8125, 51.2031) knots 0 0 0 1 2 2 2
  spline S225 degree 2 poles (11.8125, 51.2031) (11.4986, 51.2031) (10.9773, 51.4625) (10.6893, 51.945) (10.6893, 52.2044) knots 0 0 0 1 2 3 3 3
  spline S226 degree 2 poles (10.6893, 52.2044) (10.6893, 52.4845) (11.0084, 52.98) (11.6102, 53.2757) (11.9967, 53.2757) knots 0 0 0 1 2 3 3 3
  spline S227 degree 2 poles (11.9967, 53.2757) (12.4973, 53.2757) (13.4156, 52.7958) (13.9707, 51.8438) (13.994, 51.1953) knots 0 0 0 1 2 3 3 3
  spline S228 degree 2 poles (12.4532, 52.5416) (12.1912, 52.5649) (11.9915, 52.5649) knots 0 0 0 1 1 1
  spline S229 degree 2 poles (11.9915, 52.5649) (11.5661, 52.5649) (11.1978, 52.4664) knots 0 0 0 1 1 1
  spline S230 degree 2 poles (11.1978, 52.4664) (10.9954, 52.4093) (10.8994, 52.3003) knots 0 0 0 1 1 1
  spline S231 degree 2 poles (10.8994, 52.3003) (10.8476, 52.2407) (10.8476, 52.1473) knots 0 0 0 1 1 1
  spline S232 degree 2 poles (10.8476, 52.1473) (10.8476, 52.0306) (10.9487, 51.9631) knots 0 0 0 1 1 1
  spline S233 degree 2 poles (10.9487, 51.9631) (11.0862, 51.8723) (11.4753, 51.8723) knots 0 0 0 1 1 1
  spline S234 degree 2 poles (11.4753, 51.8723) (12.1238, 51.8723) (12.3702, 52.028) knots 0 0 0 1 1 1
  spline S235 degree 2 poles (12.3702, 52.028) (12.5284, 52.1291) (12.5284, 52.3003) knots 0 0 0 1 1 1
  spline S236 degree 2 poles (12.5284, 52.3003) (12.5284, 52.3911) (12.4532, 52.5416) knots 0 0 0 1 1 1
  line L127 (10.7542, 54.1758) -> (10.7542, 55.6673)
  line L128 (10.7542, 55.6673) -> (11.3586, 55.4312)
  line L129 (11.3586, 55.4312) -> (11.3586, 54.1758)
  line L130 (11.3586, 54.1758) -> (11.675, 54.059)
  spline S237 degree 2 poles (11.675, 54.059) (11.7062, 54.8684) (12.0771, 55.3041) knots 0 0 0 1 1 1
  spline S238 degree 2 poles (12.0771, 55.3041) (12.3832, 55.6621) (12.8397, 55.6621) knots 0 0 0 1 1 1
  spline S239 degree 2 poles (12.8397, 55.6621) (13.1328, 55.6621) (13.6931, 55.3301) (13.994, 54.7257) (13.994, 54.3625) knots 0 0 0 1 2 3 3 3
  spline S240 degree 2 poles (13.994, 54.3625) (13.994, 53.9734) (13.8488, 53.7659) knots 0 0 0 1 1 1
  spline S241 degree 2 poles (13.8488, 53.7659) (13.745, 53.6207) (13.6153, 53.6207) knots 0 0 0 1 1 1
  spline S242 degree 2 poles (13.6153, 53.6207) (13.5142, 53.6207) (13.3585, 53.7737) (13.3585, 53.8749) knots 0 0 0 1 2 2 2
  spline S243 degree 2 poles (13.3585, 53.8749) (13.3585, 53.9657) (13.4337, 54.1524) (13.5946, 54.3807) knots 0 0 0 1 2 2 2
  spline S244 degree 2 poles (13.5946, 54.3807) (13.6931, 54.5234) (13.7294, 54.6271) knots 0 0 0 1 1 1
  spline S245 degree 2 poles (13.7294, 54.6271) (13.758, 54.6998) (13.758, 54.7905) knots 0 0 0 1 1 1
  spline S246 degree 2 poles (13.758, 54.7905) (13.758, 54.9825) (13.4778, 55.2523) (13.2807, 55.2523) knots 0 0 0 1 2 2 2
  spline S247 degree 2 poles (13.2807, 55.2523) (12.8683, 55.2523) (12.3547, 54.4274) (12.3547, 53.7971) knots 0 0 0 1 2 2 2
  spline S248 degree 2 poles (12.3547, 53.7971) (12.3547, 53.7348) (12.3572, 53.6077) knots 0 0 0 1 1 1
  line L131 (12.3572, 53.6077) -> (10.7542, 54.1758)
  spline S249 degree 2 poles (12.3417, 58.0693) (12.8164, 58.0693) (13.2288, 57.937) knots 0 0 0 1 1 1
  spline S250 degree 2 poles (13.2288, 57.937) (13.4804, 57.8566) (13.8047, 57.5868) (13.994, 57.2444) (13.994, 57.0447) knots 0 0 0 1 2 3 3 3
  spline S251 degree 2 poles (13.994, 57.0447) (13.994, 56.8138) (13.7606, 56.4429) (13.5427, 56.3002) knots 0 0 0 1 2 2 2
  spline S252 degree 2 poles (13.5427, 56.3002) (13.3845, 56.1991) (13.1199, 56.1212) knots 0 0 0 1 1 1
  spline S253 degree 2 poles (13.1199, 56.1212) (12.7593, 56.0201) (12.378, 56.0201) knots 0 0 0 1 1 1
  spline S254 degree 2 poles (12.378, 56.0201) (11.8618, 56.0201) (11.4286, 56.1653) knots 0 0 0 1 1 1
  spline S255 degree 2 poles (11.4286, 56.1653) (11.0706, 56.2847) (10.6893, 56.7723) (10.6893, 57.0447) knots 0 0 0 1 2 2 2
  spline S256 degree 2 poles (10.6893, 57.0447) (10.6893, 57.3196) (11.0655, 57.7995) (11.3845, 57.9137) knots 0 0 0 1 2 2 2
  spline S257 degree 2 poles (11.3845, 57.9137) (11.8229, 58.0693) (12.3417, 58.0693) knots 0 0 0 1 1 1
  spline S258 degree 2 poles (12.3365, 57.3482) (11.5038, 57.3482) (11.3664, 57.3378) knots 0 0 0 1 1 1
  spline S259 degree 2 poles (11.3664, 57.3378) (11.0395, 57.3145) (10.9254, 57.2263) knots 0 0 0 1 1 1
  spline S260 degree 2 poles (10.9254, 57.2263) (10.8502, 57.1692) (10.8502, 57.0369) knots 0 0 0 1 1 1
  spline S261 degree 2 poles (10.8502, 57.0369) (10.8502, 56.9357) (10.9072, 56.8787) knots 0 0 0 1 1 1
  spline S262 degree 2 poles (10.9072, 56.8787) (10.9876, 56.7905) (11.4027, 56.7308) (12.64, 56.7308) knots 0 0 0 1 2 2 2
  spline S263 degree 2 poles (12.64, 56.7308) (13.3144, 56.7308) (13.5453, 56.7775) knots 0 0 0 1 1 1
  spline S264 degree 2 poles (13.5453, 56.7775) (13.7113, 56.8138) (13.8228, 56.9435) (13.8228, 57.0525) knots 0 0 0 1 2 2 2
  spline S265 degree 2 poles (13.8228, 57.0525) (13.8228, 57.1692) (13.7476, 57.2263) knots 0 0 0 1 1 1
  spline S266 degree 2 poles (13.7476, 57.2263) (13.6179, 57.3248) (13.343, 57.3378) knots 0 0 0 1 1 1
  line L132 (13.343, 57.3378) -> (12.3365, 57.3482)
  spline S267 degree 2 poles (12.3417, 60.4687) (12.8164, 60.4687) (13.2288, 60.3364) knots 0 0 0 1 1 1
  spline S268 degree 2 poles (13.2288, 60.3364) (13.4804, 60.256) (13.8047, 59.9862) (13.994, 59.6438) (13.994, 59.4441) knots 0 0 0 1 2 3 3 3
  spline S269 degree 2 poles (13.994, 59.4441) (13.994, 59.2132) (13.7606, 58.8423) (13.5427, 58.6996) knots 0 0 0 1 2 2 2
  spline S270 degree 2 poles (13.5427, 58.6996) (13.3845, 58.5985) (13.1199, 58.5206) knots 0 0 0 1 1 1
  spline S271 degree 2 poles (13.1199, 58.5206) (12.7593, 58.4195) (12.378, 58.4195) knots 0 0 0 1 1 1
  spline S272 degree 2 poles (12.378, 58.4195) (11.8618, 58.4195) (11.4286, 58.5647) knots 0 0 0 1 1 1
  spline S273 degree 2 poles (11.4286, 58.5647) (11.0706, 58.6841) (10.6893, 59.1717) (10.6893, 59.4441) knots 0 0 0 1 2 2 2
  spline S274 degree 2 poles (10.6893, 59.4441) (10.6893, 59.7191) (11.0655, 60.1989) (11.3845, 60.3131) knots 0 0 0 1 2 2 2
  spline S275 degree 2 poles (11.3845, 60.3131) (11.8229, 60.4687) (12.3417, 60.4687) knots 0 0 0 1 1 1
  spline S276 degree 2 poles (12.3365, 59.7476) (11.5038, 59.7476) (11.3664, 59.7372) knots 0 0 0 1 1 1
  spline S277 degree 2 poles (11.3664, 59.7372) (11.0395, 59.7139) (10.9254, 59.6257) knots 0 0 0 1 1 1
  spline S278 degree 2 poles (10.9254, 59.6257) (10.8502, 59.5686) (10.8502, 59.4363) knots 0 0 0 1 1 1
  spline S279 degree 2 poles (10.8502, 59.4363) (10.8502, 59.3352) (10.9072, 59.2781) knots 0 0 0 1 1 1
  spline S280 degree 2 poles (10.9072, 59.2781) (10.9876, 59.1899) (11.4027, 59.1302) (12.64, 59.1302) knots 0 0 0 1 2 2 2
  spline S281 degree 2 poles (12.64, 59.1302) (13.3144, 59.1302) (13.5453, 59.1769) knots 0 0 0 1 1 1
  spline S282 degree 2 poles (13.5453, 59.1769) (13.7113, 59.2132) (13.8228, 59.3429) (13.8228, 59.4519) knots 0 0 0 1 2 2 2
  spline S283 degree 2 poles (13.8228, 59.4519) (13.8228, 59.5686) (13.7476, 59.6257) knots 0 0 0 1 1 1
  spline S284 degree 2 poles (13.7476, 59.6257) (13.6179, 59.7242) (13.343, 59.7372) knots 0 0 0 1 1 1
  line L133 (13.343, 59.7372) -> (12.3365, 59.7476)
  line L134 (10.6893, 62.2067) -> (13.2859, 62.2067)
  spline S285 degree 2 poles (13.2859, 62.2067) (13.579, 62.2067) (13.7398, 62.2585) (13.8436, 62.422) (13.8436, 62.6035) knots 0 0 0 1 2 3 3 3
  line L135 (13.8436, 62.6035) -> (13.8436, 62.6762)
  line L136 (13.8436, 62.6762) -> (13.9292, 62.6762)
  line L137 (13.9292, 62.6762) -> (13.9292, 61.0031)
  line L138 (13.9292, 61.0031) -> (13.8436, 61.0031)
  line L139 (13.8436, 61.0031) -> (13.8436, 61.0861)
  spline S286 degree 2 poles (13.8436, 61.0861) (13.8436, 61.291) (13.7502, 61.4648) (13.5868, 61.5244) (13.2859, 61.5244) knots 0 0 0 1 2 3 3 3
  line L140 (13.2859, 61.5244) -> (11.6413, 61.5244)
  spline S287 degree 2 poles (11.6413, 61.5244) (11.4208, 61.5244) (11.3093, 61.4829) (11.2315, 61.3662) (11.2315, 61.291) knots 0 0 0 1 2 3 3 3
  spline S288 degree 2 poles (11.2315, 61.291) (11.2315, 61.1717) (11.3067, 61.0005) knots 0 0 0 1 1 1
  line L141 (11.3067, 61.0005) -> (11.2237, 60.959)
  line L142 (11.2237, 60.959) -> (10.6893, 62.1288)
  line L143 (10.6893, 62.1288) -> (10.6893, 62.2067)
  line L144 (15.711, 28.6253) -> (18.3076, 28.6253)
  spline S289 degree 2 poles (18.3076, 28.6253) (18.6007, 28.6253) (18.7615, 28.6772) (18.8653, 28.8406) (18.8653, 29.0222) knots 0 0 0 1 2 3 3 3
  line L145 (18.8653, 29.0222) -> (18.8653, 29.0948)
  line L146 (18.8653, 29.0948) -> (18.9509, 29.0948)
  line L147 (18.9509, 29.0948) -> (18.9509, 27.4217)
  line L148 (18.9509, 27.4217) -> (18.8653, 27.4217)
  line L149 (18.8653, 27.4217) -> (18.8653, 27.5047)
  spline S290 degree 2 poles (18.8653, 27.5047) (18.8653, 27.7097) (18.7719, 27.8835) (18.6085, 27.9431) (18.3076, 27.9431) knots 0 0 0 1 2 3 3 3
  line L150 (18.3076, 27.9431) -> (16.663, 27.9431)
  spline S291 degree 2 poles (16.663, 27.9431) (16.4425, 27.9431) (16.331, 27.9016) (16.2532, 27.7849) (16.2532, 27.7097) knots 0 0 0 1 2 3 3 3
  spline S292 degree 2 poles (16.2532, 27.7097) (16.2532, 27.5903) (16.3284, 27.4191) knots 0 0 0 1 1 1
  line L151 (16.3284, 27.4191) -> (16.2454, 27.3776)
  line L152 (16.2454, 27.3776) -> (15.711, 28.5475)
  line L153 (15.711, 28.5475) -> (15.711, 28.6253)
  spline S293 degree 2 poles (17.3634, 31.6862) (17.8381, 31.6862) (18.2505, 31.5539) knots 0 0 0 1 1 1
  spline S294 degree 2 poles (18.2505, 31.5539) (18.5021, 31.4735) (18.8264, 31.2037) (19.0157, 30.8613) (19.0157, 30.6616) knots 0 0 0 1 2 3 3 3
  spline S295 degree 2 poles (19.0157, 30.6616) (19.0157, 30.4307) (18.7823, 30.0598) (18.5644, 29.9171) knots 0 0 0 1 2 2 2
  spline S296 degree 2 poles (18.5644, 29.9171) (18.4062, 29.816) (18.1416, 29.7381) knots 0 0 0 1 1 1
  spline S297 degree 2 poles (18.1416, 29.7381) (17.781, 29.637) (17.3997, 29.637) knots 0 0 0 1 1 1
  spline S298 degree 2 poles (17.3997, 29.637) (16.8835, 29.637) (16.4503, 29.7822) knots 0 0 0 1 1 1
  spline S299 degree 2 poles (16.4503, 29.7822) (16.0924, 29.9016) (15.711, 30.3892) (15.711, 30.6616) knots 0 0 0 1 2 2 2
  spline S300 degree 2 poles (15.711, 30.6616) (15.711, 30.9365) (16.0872, 31.4164) (16.4062, 31.5306) knots 0 0 0 1 2 2 2
  spline S301 degree 2 poles (16.4062, 31.5306) (16.8446, 31.6862) (17.3634, 31.6862) knots 0 0 0 1 1 1
  spline S302 degree 2 poles (17.3582, 30.9651) (16.5256, 30.9651) (16.3881, 30.9547) knots 0 0 0 1 1 1
  spline S303 degree 2 poles (16.3881, 30.9547) (16.0612, 30.9314) (15.9471, 30.8432) knots 0 0 0 1 1 1
  spline S304 degree 2 poles (15.9471, 30.8432) (15.8719, 30.7861) (15.8719, 30.6538) knots 0 0 0 1 1 1
  spline S305 degree 2 poles (15.8719, 30.6538) (15.8719, 30.5526) (15.9289, 30.4956) knots 0 0 0 1 1 1
  spline S306 degree 2 poles (15.9289, 30.4956) (16.0094, 30.4074) (16.4244, 30.3477) (17.6617, 30.3477) knots 0 0 0 1 2 2 2
  spline S307 degree 2 poles (17.6617, 30.3477) (18.3361, 30.3477) (18.567, 30.3944) knots 0 0 0 1 1 1
  spline S308 degree 2 poles (18.567, 30.3944) (18.733, 30.4307) (18.8445, 30.5604) (18.8445, 30.6694) knots 0 0 0 1 2 2 2
  spline S309 degree 2 poles (18.8445, 30.6694) (18.8445, 30.7861) (18.7693, 30.8432) knots 0 0 0 1 1 1
  spline S310 degree 2 poles (18.7693, 30.8432) (18.6396, 30.9417) (18.3647, 30.9547) knots 0 0 0 1 1 1
  line L154 (18.3647, 30.9547) -> (17.3582, 30.9651)
  line L155 (15.9601, 32.8924) -> (16.7616, 32.8924)
  line L156 (16.7616, 32.8924) -> (16.7616, 33.4112)
  line L157 (16.7616, 33.4112) -> (16.9899, 33.4112)
  line L158 (16.9899, 33.4112) -> (16.9899, 32.8924)
  line L159 (16.9899, 32.8924) -> (18.3439, 32.8924)
  spline S311 degree 2 poles (18.3439, 32.8924) (18.5333, 32.8924) (18.6448, 32.9287) (18.7123, 33.0169) (18.7123, 33.0558) knots 0 0 0 1 2 3 3 3
  spline S312 degree 2 poles (18.7123, 33.0558) (18.7123, 33.2062) (18.4814, 33.3437) knots 0 0 0 1 1 1
  line L160 (18.4814, 33.3437) -> (18.5333, 33.4138)
  spline S313 degree 2 poles (18.5333, 33.4138) (18.982, 33.2244) (18.982, 32.7964) knots 0 0 0 1 1 1
  spline S314 degree 2 poles (18.982, 32.7964) (18.982, 32.5889) (18.7486, 32.2984) (18.6059, 32.2595) knots 0 0 0 1 2 2 2
  spline S315 degree 2 poles (18.6059, 32.2595) (18.5281, 32.2361) (18.1753, 32.2361) knots 0 0 0 1 1 1
  line L161 (18.1753, 32.2361) -> (16.9899, 32.2361)
  line L162 (16.9899, 32.2361) -> (16.9899, 31.9508)
  line L163 (16.9899, 31.9508) -> (16.9069, 31.9508)
  spline S316 degree 2 poles (16.9069, 31.9508) (16.6993, 32.2465) (16.2428, 32.6615) (15.9601, 32.8146) knots 0 0 0 1 2 2 2
  line L164 (15.9601, 32.8146) -> (15.9601, 32.8924)
  line L165 (15.7759, 34.5162) -> (17.0443, 34.5162)
  spline S317 degree 2 poles (17.0443, 34.5162) (16.855, 34.6978) (16.6968, 34.9961) (16.6968, 35.1595) knots 0 0 0 1 2 2 2
  spline S318 degree 2 poles (16.6968, 35.1595) (16.6968, 35.3644) (16.9302, 35.6575) (17.2467, 35.7535) (17.6228, 35.7535) knots 0 0 0 1 2 3 3 3
  line L166 (17.6228, 35.7535) -> (18.4762, 35.7535)
  spline S319 degree 2 poles (18.4762, 35.7535) (18.7278, 35.7535) (18.8523, 35.8469) (18.8679, 35.9896) knots 0 0 0 1 2 2 2
  line L167 (18.8679, 35.9896) -> (18.9509, 35.9896)
  line L168 (18.9509, 35.9896) -> (18.9509, 34.8794)
  line L169 (18.9509, 34.8794) -> (18.8679, 34.8794)
  spline S320 degree 2 poles (18.8679, 34.8794) (18.8523, 34.9961) (18.7745, 35.0557) knots 0 0 0 1 1 1
  spline S321 degree 2 poles (18.7745, 35.0557) (18.7123, 35.0972) (18.4762, 35.0972) knots 0 0 0 1 1 1
  line L170 (18.4762, 35.0972) -> (17.5009, 35.0972)
  spline S322 degree 2 poles (17.5009, 35.0972) (17.2285, 35.0972) (17.091, 35.0557) (17.0132, 34.9546) (17.0132, 34.8923) knots 0 0 0 1 2 3 3 3
  spline S323 degree 2 poles (17.0132, 34.8923) (17.0132, 34.7963) (17.1429, 34.62) (17.3037, 34.5162) knots 0 0 0 1 2 2 2
  line L171 (17.3037, 34.5162) -> (18.4762, 34.5162)
  spline S324 degree 2 poles (18.4762, 34.5162) (18.7097, 34.5162) (18.7693, 34.5525) knots 0 0 0 1 1 1
  spline S325 degree 2 poles (18.7693, 34.5525) (18.8497, 34.5966) (18.8679, 34.7341) knots 0 0 0 1 1 1
  line L172 (18.8679, 34.7341) -> (18.9509, 34.7341)
  line L173 (18.9509, 34.7341) -> (18.9509, 33.6239)
  line L174 (18.9509, 33.6239) -> (18.8679, 33.6239)
  spline S326 degree 2 poles (18.8679, 33.6239) (18.8549, 33.7614) (18.7797, 33.821) knots 0 0 0 1 1 1
  spline S327 degree 2 poles (18.7797, 33.821) (18.7278, 33.8599) (18.4762, 33.8599) knots 0 0 0 1 1 1
  line L175 (18.4762, 33.8599) -> (16.2506, 33.8599)
  spline S328 degree 2 poles (16.2506, 33.8599) (16.0016, 33.8599) (15.8797, 33.7691) (15.8615, 33.6239) knots 0 0 0 1 2 2 2
  line L176 (15.8615, 33.6239) -> (15.7759, 33.6239)
  line L177 (15.7759, 33.6239) -> (15.7759, 34.5162)
  line L178 (15.7033, 39.577) -> (16.7616, 39.6029)
  line L179 (16.7616, 39.6029) -> (16.7616, 39.507)
  spline S329 degree 2 poles (16.7616, 39.507) (16.3647, 39.4395) (15.8797, 38.9052) (15.8797, 38.5965) knots 0 0 0 1 2 2 2
  spline S330 degree 2 poles (15.8797, 38.5965) (15.8797, 38.3578) (16.1339, 38.0777) (16.2999, 38.0777) knots 0 0 0 1 2 2 2
  spline S331 degree 2 poles (16.2999, 38.0777) (16.4062, 38.0777) (16.4866, 38.127) knots 0 0 0 1 1 1
  spline S332 degree 2 poles (16.4866, 38.127) (16.5982, 38.1944) (16.7045, 38.3449) knots 0 0 0 1 1 1
  spline S333 degree 2 poles (16.7045, 38.3449) (16.7824, 38.4564) (16.9795, 38.8559) knots 0 0 0 1 1 1
  spline S334 degree 2 poles (16.9795, 38.8559) (17.2519, 39.4136) (17.4957, 39.6081) knots 0 0 0 1 1 1
  spline S335 degree 2 poles (17.4957, 39.6081) (17.7395, 39.8001) (18.0534, 39.8001) knots 0 0 0 1 1 1
  spline S336 degree 2 poles (18.0534, 39.8001) (18.4503, 39.8001) (19.0235, 39.1801) (19.0235, 38.7002) knots 0 0 0 1 2 2 2
  spline S337 degree 2 poles (19.0235, 38.7002) (19.0235, 38.5498) (18.9639, 38.2826) (18.8783, 38.0829) knots 0 0 0 1 2 2 2
  spline S338 degree 2 poles (18.8783, 38.0829) (18.8316, 37.9687) (18.8316, 37.8961) knots 0 0 0 1 1 1
  spline S339 degree 2 poles (18.8316, 37.8961) (18.8316, 37.8365) (18.9276, 37.699) (19.0235, 37.6575) knots 0 0 0 1 2 2 2
  line L180 (19.0235, 37.6575) -> (19.0235, 37.5719)